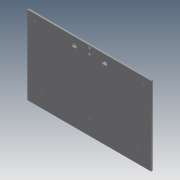
# Autodesk Inventor part: it bottom
Saved by Autodesk Inventor 2011 (Build 150239000, 239)
## iProperties
Created: 2011-09-03
Part Number: it bottom
Document SubType Name: Modeling
Designer: Matthew
Density: 1 g/cm^3
Author: Matthew
Autodesk Inventor part; units mm, degrees
ref_plane "YZ Plane" through (0, 0, 0) normal (1, 0, 0) x (0, 1, 0)
ref_plane "XZ Plane" through (0, 0, 0) normal (0, 1, 0) x (-1, 0, 0)
ref_plane "XY Plane" through (0, 0, 0) normal (0, 0, 1) x (1, 0, 0)
sketch "Sketch1" plane through (0, 0, 0) normal (0, 0, 1) x (1, 0, 0)
  line L0 (-37.7036, 22.272) -> (457.5964, 22.272)
  line L1 (457.5964, 22.272) -> (457.5964, -304.118)
  line L2 (457.5964, -304.118) -> (-37.7036, -304.118)
  line L3 (-37.7036, -304.118) -> (-37.7036, 22.272)
  point P0 (0, 0)
  dimension "d0" = 495.3
  dimension "d1" = 326.39
  constraints: 8 end point, 2 parallel, 1 horizontal, 1 perpendicular
  measures "d0" distance of L1.end L2.end
  measures "d1" distance of L0.end L1.end
extrude "Extrusion1" add sketch "Sketch1" along normal blind 6.35
sketch "Sketch2" plane through (0, 0, 6.35) normal (0, 0, 1) x (1, 0, 0)
  line L0 (-37.7036, 22.272) -> (457.5964, 22.272) projected
  line L1 (-37.7036, 22.272) -> (-18.6536, 22.272)
  line L2 (-18.6536, 22.272) -> (-18.6536, 15.922)
  line L3 (-18.6536, 15.922) -> (-37.7036, 15.922)
  line L4 (-37.7036, 15.922) -> (-37.7036, 22.272)
  line L5 (-18.6536, 15.922) -> (32.1464, 15.922)
  line L6 (32.1464, 15.922) -> (32.1464, 22.272)
  line L7 (32.1464, 22.272) -> (-18.6536, 22.272)
  line L8 (-18.6536, 22.272) -> (-18.6536, 15.922)
  line L9 (32.1464, 15.922) -> (82.9464, 15.922)
  line L10 (82.9464, 15.922) -> (82.9464, 22.272)
  line L11 (82.9464, 22.272) -> (32.1464, 22.272)
  line L12 (32.1464, 22.272) -> (32.1464, 15.922)
  line L13 (82.9464, 15.922) -> (133.7464, 15.922)
  line L14 (133.7464, 15.922) -> (133.7464, 22.272)
  line L15 (133.7464, 22.272) -> (82.9464, 22.272)
  line L16 (82.9464, 22.272) -> (82.9464, 15.922)
  line L17 (133.7464, 15.922) -> (184.5464, 15.922)
  line L18 (184.5464, 15.922) -> (184.5464, 22.272)
  line L19 (184.5464, 22.272) -> (133.7464, 22.272)
  line L20 (133.7464, 22.272) -> (133.7464, 15.922)
  line L21 (184.5464, 15.922) -> (235.3464, 15.922)
  line L22 (235.3464, 15.922) -> (235.3464, 22.272)
  line L23 (235.3464, 22.272) -> (184.5464, 22.272)
  line L24 (184.5464, 22.272) -> (184.5464, 15.922)
  line L25 (235.3464, 15.922) -> (286.1464, 15.922)
  line L26 (286.1464, 15.922) -> (286.1464, 22.272)
  line L27 (286.1464, 22.272) -> (235.3464, 22.272)
  line L28 (235.3464, 22.272) -> (235.3464, 15.922)
  line L29 (286.1464, 15.922) -> (336.9464, 15.922)
  line L30 (336.9464, 15.922) -> (336.9464, 22.272)
  line L31 (336.9464, 22.272) -> (286.1464, 22.272)
  line L32 (286.1464, 22.272) -> (286.1464, 15.922)
  line L33 (336.9464, 15.922) -> (387.7464, 15.922)
  line L34 (387.7464, 15.922) -> (387.7464, 22.272)
  line L35 (387.7464, 22.272) -> (336.9464, 22.272)
  line L36 (336.9464, 22.272) -> (336.9464, 15.922)
  line L37 (387.7464, 15.922) -> (438.5464, 15.922)
  line L38 (438.5464, 15.922) -> (438.5464, 22.272)
  line L39 (438.5464, 22.272) -> (387.7464, 22.272)
  line L40 (387.7464, 22.272) -> (387.7464, 15.922)
  line L41 (438.5464, 15.922) -> (457.5964, 15.922)
  line L42 (457.5964, 15.922) -> (457.5964, 22.272)
  line L43 (457.5964, 22.272) -> (438.5464, 22.272)
  line L44 (438.5464, 22.272) -> (438.5464, 15.922)
  point P0 (0, 0)
  dimension "d4" = 19.05
  dimension "d5" = 6.35
  dimension "d6" = 50.8
  dimension "d7" = 50.8
  dimension "d8" = 50.8
  dimension "d9" = 50.8
  dimension "d10" = 50.8
  dimension "d11" = 50.8
  dimension "d12" = 50.8
  dimension "d13" = 50.8
  dimension "d14" = 50.8
  constraints: 88 end point, 22 parallel, 11 horizontal, 11 perpendicular, 10 other
  measures "d4" distance of L2.end L3.end
  measures "d5" distance of L1.end L2.end
  measures "d6" distance of L7.end L6.end
  measures "d7" distance of L11.end L10.end
  measures "d8" distance of L15.end L14.end
  measures "d9" distance of L19.end L18.end
  measures "d10" distance of L23.end L22.end
  measures "d11" distance of L27.end L26.end
  measures "d12" distance of L31.end L30.end
  measures "d13" distance of L35.end L34.end
  measures "d14" distance of L39.end L38.end
extrude "Extrusion2" cut sketch "Sketch2" against normal blind 6.35 contours L0 L2 L3 L4 | L0 L10 L9 L6 | L0 L18 L17 L14 | L0 L26 L25 L22 | L0 L34 L33 L30 | L0 L42 L41 L38
sketch "Sketch3" plane through (0, 0, 6.35) normal (0, 0, 1) x (1, 0, 0)
  line L0 (457.5964, -304.118) -> (-37.7036, -304.118) projected
  line L1 (-37.7036, -304.118) -> (-18.6536, -304.118)
  line L2 (-18.6536, -304.118) -> (-18.6536, -297.768)
  line L3 (-18.6536, -297.768) -> (-37.7036, -297.768)
  line L4 (-37.7036, -297.768) -> (-37.7036, -304.118)
  line L5 (-18.6536, -297.768) -> (32.1464, -297.768)
  line L6 (32.1464, -297.768) -> (32.1464, -304.118)
  line L7 (32.1464, -304.118) -> (-18.6536, -304.118)
  line L8 (-18.6536, -304.118) -> (-18.6536, -297.768)
  line L9 (32.1464, -304.118) -> (82.9464, -304.118)
  line L10 (82.9464, -304.118) -> (82.9464, -297.768)
  line L11 (82.9464, -297.768) -> (32.1464, -297.768)
  line L12 (32.1464, -297.768) -> (32.1464, -304.118)
  line L13 (82.9464, -297.768) -> (133.7464, -297.768)
  line L14 (133.7464, -297.768) -> (133.7464, -304.118)
  line L15 (133.7464, -304.118) -> (82.9464, -304.118)
  line L16 (82.9464, -304.118) -> (82.9464, -297.768)
  line L17 (133.7464, -297.768) -> (184.5464, -297.768)
  line L18 (184.5464, -297.768) -> (184.5464, -304.118)
  line L19 (184.5464, -304.118) -> (133.7464, -304.118)
  line L20 (133.7464, -304.118) -> (133.7464, -297.768)
  line L21 (184.5464, -297.768) -> (235.3464, -297.768)
  line L22 (235.3464, -297.768) -> (235.3464, -304.118)
  line L23 (235.3464, -304.118) -> (184.5464, -304.118)
  line L24 (184.5464, -304.118) -> (184.5464, -297.768)
  line L25 (235.3464, -304.118) -> (286.1464, -304.118)
  line L26 (286.1464, -304.118) -> (286.1464, -297.768)
  line L27 (286.1464, -297.768) -> (235.3464, -297.768)
  line L28 (235.3464, -297.768) -> (235.3464, -304.118)
  line L29 (286.1464, -297.768) -> (336.9464, -297.768)
  line L30 (336.9464, -297.768) -> (336.9464, -304.118)
  line L31 (336.9464, -304.118) -> (286.1464, -304.118)
  line L32 (286.1464, -304.118) -> (286.1464, -297.768)
  line L33 (336.9464, -297.768) -> (387.7464, -297.768)
  line L34 (387.7464, -297.768) -> (387.7464, -304.118)
  line L35 (387.7464, -304.118) -> (336.9464, -304.118)
  line L36 (336.9464, -304.118) -> (336.9464, -297.768)
  line L37 (387.7464, -297.768) -> (438.5464, -297.768)
  line L38 (438.5464, -297.768) -> (438.5464, -304.118)
  line L39 (438.5464, -304.118) -> (387.7464, -304.118)
  line L40 (387.7464, -304.118) -> (387.7464, -297.768)
  line L41 (438.5464, -297.768) -> (457.5964, -297.768)
  line L42 (457.5964, -297.768) -> (457.5964, -304.118)
  line L43 (457.5964, -304.118) -> (438.5464, -304.118)
  line L44 (438.5464, -304.118) -> (438.5464, -297.768)
  point P0 (0, 0)
  dimension "d17" = 19.05
  dimension "d18" = 6.35
  constraints: 88 end point, 22 parallel, 11 horizontal, 11 perpendicular, 8 other
  measures "d17" distance of L3.end L2.end
  measures "d18" distance of L2.end L1.end
extrude "Extrusion3" cut sketch "Sketch3" against normal blind 6.35 contours L0 L38 L41 L42 | L0 L30 L33 L34 | L0 L14 L17 L18 | L0 L6 L11 L10 | L0 L4 L3 L2
sketch "Sketch4" plane through (0, 0, 6.35) normal (0, 0, 1) x (1, 0, 0)
  line L0 (336.9464, -304.118) -> (184.5464, -304.118) projected
  line L1 (184.5464, -304.118) -> (235.3464, -304.118)
  line L2 (235.3464, -304.118) -> (286.1464, -304.118)
  line L3 (286.1464, -304.118) -> (286.1464, -297.768)
  line L4 (286.1464, -297.768) -> (235.3464, -297.768)
  line L5 (235.3464, -297.768) -> (235.3464, -304.118)
  point P0 (0, 0)
  dimension "d21" = 50.8
  dimension "d22" = 50.8
  constraints: 10 end point, 2 parallel, 1 horizontal, 1 perpendicular, 1 point on line
  measures "d21" distance of L0.end L1.end
  measures "d22" distance of L4.end L3.end
extrude "Extrusion4" cut sketch "Sketch4" against normal blind 6.35
sketch "Sketch5" plane through (0, 0, 6.35) normal (0, 0, 1) x (1, 0, 0)
  line L0 (457.5964, 15.922) -> (457.5964, -297.768) projected
  line L1 (-37.7036, -297.768) -> (-37.7036, 15.922) projected
  line L2 (-37.7036, -297.768) -> (-18.6536, -297.768) projected
  line L3 (457.5964, 15.922) -> (457.5964, -166.323)
  line L4 (457.5964, -166.323) -> (451.2464, -166.323)
  line L5 (451.2464, -166.323) -> (451.2464, -115.523)
  line L6 (451.2464, -115.523) -> (457.5964, -115.523)
  line L7 (457.5964, -115.523) -> (457.5964, -166.323)
  line L8 (451.2464, -115.523) -> (457.5964, -115.523)
  line L9 (457.5964, -115.523) -> (457.5964, -64.723)
  line L10 (457.5964, -64.723) -> (451.2464, -64.723)
  line L11 (451.2464, -64.723) -> (451.2464, -115.523)
  line L12 (451.2464, -64.723) -> (457.5964, -64.723)
  line L13 (457.5964, -64.723) -> (457.5964, -13.923)
  line L14 (457.5964, -13.923) -> (451.2464, -13.923)
  line L15 (451.2464, -13.923) -> (451.2464, -64.723)
  line L16 (451.2464, -166.323) -> (457.5964, -166.323)
  line L17 (457.5964, -166.323) -> (457.5964, -217.123)
  line L18 (457.5964, -217.123) -> (451.2464, -217.123)
  line L19 (451.2464, -217.123) -> (451.2464, -166.323)
  line L20 (451.2464, -217.123) -> (457.5964, -217.123)
  line L21 (457.5964, -217.123) -> (457.5964, -267.923)
  line L22 (457.5964, -267.923) -> (451.2464, -267.923)
  line L23 (451.2464, -267.923) -> (451.2464, -217.123)
  line L24 (451.2464, -267.923) -> (457.5964, -267.923)
  line L25 (457.5964, -267.923) -> (457.5964, -297.768)
  line L26 (457.5964, -297.768) -> (451.2464, -297.768)
  line L27 (451.2464, -297.768) -> (451.2464, -267.923)
  line L28 (451.2464, -13.923) -> (457.5964, -13.923)
  line L29 (457.5964, -13.923) -> (457.5964, 15.922)
  line L30 (457.5964, 15.922) -> (451.2464, 15.922)
  line L31 (451.2464, 15.922) -> (451.2464, -13.923)
  line L32 (-37.7036, 15.922) -> (-31.3536, 15.922)
  line L33 (-31.3536, 15.922) -> (-31.3536, -13.923)
  line L34 (-31.3536, -13.923) -> (-37.7036, -13.923)
  line L35 (-37.7036, -13.923) -> (-37.7036, 15.922)
  line L36 (-37.7036, -64.723) -> (-31.3536, -64.723)
  line L37 (-31.3536, -64.723) -> (-31.3536, -115.523)
  line L38 (-31.3536, -115.523) -> (-37.7036, -115.523)
  line L39 (-37.7036, -115.523) -> (-37.7036, -64.723)
  line L40 (-37.7036, -166.323) -> (-31.3536, -166.323)
  line L41 (-31.3536, -166.323) -> (-31.3536, -217.123)
  line L42 (-31.3536, -217.123) -> (-37.7036, -217.123)
  line L43 (-37.7036, -217.123) -> (-37.7036, -166.323)
  line L44 (-37.7036, -267.923) -> (-31.3536, -267.923)
  line L45 (-31.3536, -267.923) -> (-31.3536, -297.768)
  line L46 (-31.3536, -297.768) -> (-37.7036, -297.768)
  line L47 (-37.7036, -297.768) -> (-37.7036, -267.923)
  point P0 (0, 0)
  dimension "d25" = 182.245
  dimension "d26" = 6.35
  dimension "d27" = 50.8
  dimension "d28" = 50.8
  dimension "d29" = 50.8
  dimension "d30" = 50.8
  dimension "d31" = 50.8
  dimension "d32" = 6.35
  constraints: 90 end point, 22 parallel, 11 horizontal, 11 perpendicular, 9 point on line
  measures "d25" distance of L0.start L3.end
  measures "d26" distance of L5.end L6.end
  measures "d27" distance of L4.end L5.end
  measures "d28" distance of L9.end L8.end
  measures "d29" distance of L13.end L12.end
  measures "d30" distance of L16.end L17.end
  measures "d31" distance of L20.end L21.end
  measures "d32" distance of L33.end L34.end
extrude "Extrusion5" cut sketch "Sketch5" against normal blind 6.35 contours L0 L14 L31 L30 | L0 L18 L19 L4 | L0 L26 L27 L22 | L1 L44 L45 L2 | L1 L40 L41 L42 | L1 L36 L37 L38 | L1 L32 L33 L34
sketch "Sketch6" plane through (0, 0, 6.35) normal (0, 0, 1) x (1, 0, 0)
  line L0 (457.5964, -13.923) -> (457.5964, -166.323) projected
  line L1 (457.5964, -13.923) -> (457.5964, -64.723)
  line L2 (457.5964, -64.723) -> (451.2464, -64.723)
  line L3 (451.2464, -64.723) -> (451.2464, -115.523)
  line L4 (451.2464, -115.523) -> (457.5964, -115.523)
  line L5 (457.5964, -115.523) -> (457.5964, -64.723)
  point P0 (0, 0)
  constraints: 10 end point, 2 parallel, 1 horizontal, 1 perpendicular, 1 point on line
extrude "Extrusion6" cut sketch "Sketch6" against normal blind 6.35
sketch "Sketch7" plane through (0, 0, 6.35) normal (0, 0, 1) x (1, 0, 0)
  line L0 (451.2464, -13.923) -> (451.2464, 15.922) projected
  line L1 (387.7464, 15.922) -> (336.9464, 15.922) projected
  line L2 (82.9464, 15.922) -> (32.1464, 15.922) projected
  line L3 (-31.3536, 15.922) -> (-31.3536, -13.923) projected
  line L4 (451.2464, -115.523) -> (451.2464, -64.723) projected
  line L5 (-31.3536, -6.7444) -> (44.8464, -6.7444)
  line L6 (44.8464, -6.7444) -> (44.8464, 15.922)
  line L7 (44.8464, 15.922) -> (44.8464, -60.278)
  line L8 (451.2464, -6.7444) -> (375.0464, -6.7444)
  line L9 (375.0464, -6.7444) -> (375.0464, 15.922)
  line L10 (375.0464, 15.922) -> (375.0464, -60.278)
  circle A0 centre (44.8464, -60.278) radius 25.4
  circle A1 centre (375.0464, -60.278) radius 25.4
  point P0 (0, 0)
  dimension "d37" = 76.2
  dimension "d38" = 76.2
  dimension "d39" = 76.2
  dimension "d40" = 76.2
  dimension "d41" = 50.8
  dimension "d42" = 50.8
  constraints: 12 end point, 4 perpendicular, 4 point on line, 2 centre point, 2 coincident, 2 collinear
  measures "d37" distance of L5.start L5.end
  measures "d38" distance of L6.end L7.end
  measures "d39" distance of L8.start L8.end
  measures "d40" distance of L9.end L10.end
  measures "d41" diameter of A0
  measures "d42" diameter of A1
extrude "Extrusion7" cut sketch "Sketch7" against normal blind 25.4
sketch "Sketch8" plane through (0, 0, 6.35) normal (0, 0, 1) x (1, 0, 0)
  line L0 (-31.3536, -297.768) -> (-37.7036, -297.768)
  line L1 (-37.7036, -297.768) -> (-37.7036, 15.922)
  line L2 (-37.7036, 15.922) -> (-31.3536, 15.922)
  line L3 (-31.3536, 15.922) -> (-31.3536, -297.768)
  point P0 (0, 0)
  constraints: 8 end point, 2 parallel, 1 horizontal, 1 perpendicular
extrude "Extrusion8" add sketch "Sketch8" against normal blind 6.35
sketch "Sketch9" plane through (0, 0, 6.35) normal (0, 0, 1) x (1, 0, 0)
  line L0 (451.2464, -297.768) -> (457.5964, -297.768)
  line L1 (457.5964, -297.768) -> (457.5964, 15.922)
  line L2 (457.5964, 15.922) -> (451.2464, 15.922)
  line L3 (451.2464, 15.922) -> (451.2464, -297.768)
  point P0 (0, 0)
  constraints: 8 end point, 2 parallel, 1 horizontal, 1 perpendicular
extrude "Extrusion9" add sketch "Sketch9" against normal blind 6.35
sketch "Sketch10" plane through (0, 0, 6.35) normal (0, 0, 1) x (1, 0, 0)
  line L0 (457.5964, 15.922) -> (438.5464, 15.922) projected
  line L1 (438.5464, 15.922) -> (438.5464, 22.272) projected
  line L2 (387.7464, 22.272) -> (438.5464, 22.272) projected
  line L3 (387.7464, 22.272) -> (387.7464, 15.922) projected
  line L4 (387.7464, 15.922) -> (336.9464, 15.922) projected
  line L5 (336.9464, 15.922) -> (336.9464, 22.272) projected
  line L6 (286.1464, 22.272) -> (336.9464, 22.272) projected
  line L7 (286.1464, 22.272) -> (286.1464, 15.922) projected
  line L8 (286.1464, 15.922) -> (235.3464, 15.922) projected
  line L9 (235.3464, 15.922) -> (235.3464, 22.272) projected
  line L10 (184.5464, 22.272) -> (235.3464, 22.272) projected
  line L11 (184.5464, 22.272) -> (184.5464, 15.922) projected
  line L12 (184.5464, 15.922) -> (133.7464, 15.922) projected
  line L13 (133.7464, 15.922) -> (133.7464, 22.272) projected
  line L14 (82.9464, 22.272) -> (133.7464, 22.272) projected
  line L15 (82.9464, 22.272) -> (82.9464, 15.922) projected
  line L16 (82.9464, 15.922) -> (32.1464, 15.922) projected
  line L17 (32.1464, 15.922) -> (32.1464, 22.272) projected
  line L18 (-18.6536, 22.272) -> (32.1464, 22.272) projected
  line L19 (-18.6536, 22.272) -> (-18.6536, 15.922) projected
  line L20 (-18.6536, 15.922) -> (-37.7036, 15.922) projected
  line L21 (-37.7036, 15.922) -> (-37.7036, -297.768) projected
  line L22 (-37.7036, -297.768) -> (-18.6536, -297.768) projected
  line L23 (-18.6536, -297.768) -> (-18.6536, -304.118) projected
  line L24 (32.1464, -304.118) -> (-18.6536, -304.118) projected
  line L25 (32.1464, -304.118) -> (32.1464, -297.768) projected
  line L26 (32.1464, -297.768) -> (82.9464, -297.768) projected
  line L27 (82.9464, -297.768) -> (82.9464, -304.118) projected
  line L28 (133.7464, -304.118) -> (82.9464, -304.118) projected
  line L29 (133.7464, -304.118) -> (133.7464, -297.768) projected
  line L30 (133.7464, -297.768) -> (184.5464, -297.768) projected
  line L31 (184.5464, -297.768) -> (184.5464, -304.118) projected
  line L32 (235.3464, -304.118) -> (184.5464, -304.118) projected
  line L33 (235.3464, -304.118) -> (235.3464, -297.768) projected
  line L34 (235.3464, -297.768) -> (286.1464, -297.768) projected
  line L35 (286.1464, -297.768) -> (286.1464, -304.118) projected
  line L36 (336.9464, -304.118) -> (286.1464, -304.118) projected
  line L37 (336.9464, -304.118) -> (336.9464, -297.768) projected
  line L38 (336.9464, -297.768) -> (387.7464, -297.768) projected
  line L39 (387.7464, -297.768) -> (387.7464, -304.118) projected
  line L40 (438.5464, -304.118) -> (387.7464, -304.118) projected
  line L41 (438.5464, -304.118) -> (438.5464, -297.768) projected
  line L42 (438.5464, -297.768) -> (457.5964, -297.768) projected
  line L43 (457.5964, 15.922) -> (457.5964, -297.768) projected
  line L44 (-18.6536, -297.768) -> (438.5464, -297.768)
  line L45 (438.5464, 15.922) -> (-18.6536, 15.922)
  point P0 (0, 0)
  constraints: 4 end point, 1 parallel, 1 perpendicular
extrude "Extrusion10" cut sketch "Sketch10" against normal blind 6.35 contours L45 L3 L2 L1 | L41 L40 L39 L44 | L45 L7 L6 L5 | L37 L36 L35 L44 | L45 L11 L10 L9 | L33 L32 L31 L44 | L45 L15 L14 L13 | L29 L28 L27 L44 | L45 L19 L18 L17 | L25 L24 L23 L44
sketch "Sketch12" plane through (0, 0, 6.35) normal (0, 0, 1) x (1, 0, 0)
  circle A0 centre (44.8464, -60.278) radius 25.4 projected
  circle A1 centre (375.0464, -60.278) radius 25.4 projected
  point P0 (0, 0)
extrude "Extrusion11" add sketch "Sketch12" against normal blind 6.35
sketch "Sketch13" plane through (0, 0, 6.35) normal (0, 0, 1) x (1, 0, 0)
  line L0 (457.5964, 15.922) -> (-37.7036, 15.922) projected
  line L1 (-37.7036, 15.922) -> (-37.7036, -297.768) projected
  line L2 (457.5964, 15.922) -> (368.6964, 15.922)
  line L3 (368.6964, 15.922) -> (368.6964, -66.628)
  line L4 (-37.7036, -66.628) -> (44.8464, -66.628)
  circle A0 centre (368.6964, -66.628) radius 25.4
  circle A1 centre (44.8464, -66.628) radius 25.4
  point P0 (0, 0)
  dimension "d53" = 88.9
  dimension "d54" = 82.55
  dimension "d55" = 82.55
  dimension "d56" = 50.8
  dimension "d57" = 50.8
  constraints: 6 end point, 2 centre point, 2 coincident, 2 perpendicular, 2 point on line
  measures "d53" distance of L0.start L2.end
  measures "d54" distance of L2.end L3.end
  measures "d55" distance of L4.start L4.end
  measures "d56" diameter of A0
  measures "d57" diameter of A1
extrude "Extrusion12" cut sketch "Sketch13" against normal blind 6.35
sketch "Sketch14" plane through (0, 0, 6.35) normal (0, 0, 1) x (1, 0, 0)
  circle A0 centre (368.6964, -66.628) radius 25.4 projected
  circle A1 centre (44.8464, -66.628) radius 25.4 projected
  point P0 (0, 0)
extrude "Extrusion13" add sketch "Sketch14" against normal blind 6.35
sketch "Sketch15" plane through (0, 0, 6.35) normal (0, 0, 1) x (1, 0, 0)
  line L0 (457.5964, 15.922) -> (375.0464, 15.922)
  line L1 (375.0464, 15.922) -> (375.0464, -71.4032)
  line L2 (375.0464, -71.4032) -> (457.5964, -71.4032)
  line L3 (457.5964, -71.4032) -> (457.5964, 15.922)
  line L4 (-37.7036, 15.922) -> (44.8464, 15.922)
  line L5 (44.8464, 15.922) -> (44.8464, -71.4032)
  line L6 (44.8464, -71.4032) -> (-37.7036, -71.4032)
  line L7 (-37.7036, -71.4032) -> (-37.7036, 15.922)
  circle A0 centre (375.0464, -71.4032) radius 25.4
  circle A1 centre (44.8464, -71.4032) radius 25.4
  point P0 (0, 0)
  dimension "d62" = 82.55
  dimension "d63" = 87.3252
  dimension "d64" = 82.55
  dimension "d65" = 87.3252
  dimension "d66" = 50.8
  dimension "d67" = 50.8
  constraints: 16 end point, 4 parallel, 2 centre point, 2 coincident, 2 horizontal, 2 perpendicular
  measures "d62" distance of L2.end L1.end
  measures "d63" distance of L1.end L0.end
  measures "d64" distance of L5.end L6.end
  measures "d65" distance of L4.end L5.end
  measures "d66" diameter of A0
  measures "d67" diameter of A1
extrude "Extrusion14" cut sketch "Sketch15" against normal blind 6.35 contours A0 L2 L1 | L1 L2 A0 | A1 L6 L5 | L5 L6 A1
sketch "Sketch16" plane through (0, 0, 6.35) normal (0, 0, 1) x (1, 0, 0)
  line L0 (-37.7036, 15.922) -> (-5.9536, 15.922)
  line L1 (-5.9536, 15.922) -> (-5.9536, -9.478)
  line L2 (-5.9536, -9.478) -> (-37.7036, -9.478)
  line L3 (-37.7036, -9.478) -> (-37.7036, 15.922)
  line L4 (-37.7036, -297.768) -> (19.4464, -297.768)
  line L5 (19.4464, -297.768) -> (19.4464, -240.618)
  line L6 (19.4464, -240.618) -> (-37.7036, -240.618)
  line L7 (-37.7036, -240.618) -> (-37.7036, -297.768)
  line L8 (457.5964, 15.922) -> (425.8464, 15.922)
  line L9 (425.8464, 15.922) -> (425.8464, -9.478)
  line L10 (425.8464, -9.478) -> (457.5964, -9.478)
  line L11 (457.5964, -9.478) -> (457.5964, 15.922)
  line L12 (457.5964, -297.768) -> (400.4464, -297.768)
  line L13 (400.4464, -297.768) -> (400.4464, -240.618)
  line L14 (400.4464, -240.618) -> (457.5964, -240.618)
  line L15 (457.5964, -240.618) -> (457.5964, -297.768)
  circle A0 centre (400.4464, -240.618) radius 1.9812
  circle A1 centre (19.4464, -240.618) radius 1.9812
  circle A2 centre (-5.9536, -9.478) radius 1.9812
  circle A3 centre (425.8464, -9.478) radius 1.9812
  point P0 (0, 0)
  dimension "d70" = 31.75
  dimension "d71" = 25.4
  dimension "d72" = 57.15
  dimension "d73" = 57.15
  dimension "d74" = 31.75
  dimension "d75" = 57.15
  dimension "d76" = 3.9624
  dimension "d77" = 3.9624
  dimension "d78" = 3.9624
  dimension "d79" = 3.9624
  constraints: 32 end point, 8 parallel, 4 centre point, 4 coincident, 4 horizontal, 4 perpendicular
  measures "d70" distance of L1.end L2.end
  measures "d71" distance of L0.end L1.end
  measures "d72" distance of L6.end L5.end
  measures "d73" distance of L5.end L4.end
  measures "d74" distance of L10.end L9.end
  measures "d75" distance of L13.end L14.end
  measures "d76" diameter of A0
  measures "d77" diameter of A1
  measures "d78" diameter of A2
  measures "d79" diameter of A3
extrude "Extrusion15" cut sketch "Sketch16" against normal blind 25.4 contours A2 L2 L1 | L1 L2 A2 | A3 L10 L9 | L9 L10 A3
sketch "Sketch17" plane through (0, 0, 6.35) normal (0, 0, 1) x (1, 0, 0)
  circle A0 centre (425.8464, -9.478) radius 1.9812 projected
  line L0 (457.5964, 15.922) -> (457.5964, -297.768) projected
  line L1 (425.8464, -9.478) -> (425.8464, -272.368)
  line L2 (425.8464, -272.368) -> (0, -272.368)
  line L3 (0, -272.368) -> (25.4, -272.368)
  line L4 (25.4, -272.368) -> (25.4, -246.968)
  line L5 (425.8464, -246.968) -> (400.4464, -246.968)
  circle A1 centre (400.4464, -246.968) radius 1.9812
  circle A2 centre (25.4, -246.968) radius 1.9812
  point P0 (0, 0)
  dimension "d82" = 262.89
  dimension "d83" = 25.4
  dimension "d84" = 25.4
  dimension "d85" = 25.4
  dimension "d86" = 3.9624
  dimension "d87" = 3.9624
  constraints: 10 end point, 3 perpendicular, 2 centre point, 2 coincident, 2 point on line, 1 parallel
  measures "d82" distance of L1.start L1.end
  measures "d83" distance of L2.end L3.end
  measures "d84" distance of L3.end L4.end
  measures "d85" distance of L5.start L5.end
  measures "d86" diameter of A1
  measures "d87" diameter of A2
extrude "Extrusion16" cut sketch "Sketch17" against normal blind 25.4 contours A1 | A2
sketch "Sketch18" plane through (0, 0, 6.35) normal (0, 0, 1) x (1, 0, 0)
  circle A0 centre (25.4, -246.968) radius 1.9812 projected
  point P0 (0, 0)
extrude "Extrusion17" add sketch "Sketch18" against normal blind 6.35
sketch "Sketch19" plane through (0, 0, 6.35) normal (0, 0, 1) x (1, 0, 0)
  circle A0 centre (-5.9536, -9.478) radius 1.9812 projected
  line L0 (457.5964, 15.922) -> (457.5964, -297.768) projected
  line L1 (-5.9536, -9.478) -> (-5.9536, -272.368)
  line L2 (-5.9536, -272.368) -> (19.4464, -272.368)
  line L3 (19.4464, -272.368) -> (19.4464, -246.968)
  circle A1 centre (19.4464, -246.968) radius 1.9812
  point P0 (0, 0)
  dimension "d92" = 262.89
  dimension "d93" = 25.4
  dimension "d94" = 25.4
  dimension "d95" = 3.9624
  constraints: 6 end point, 2 parallel, 1 centre point, 1 coincident, 1 perpendicular
  measures "d92" distance of L1.start L1.end
  measures "d93" distance of L1.end L2.end
  measures "d94" distance of L2.end L3.end
  measures "d95" diameter of A1
extrude "Extrusion18" cut sketch "Sketch19" against normal blind 6.35 contours A1
sketch "Sketch20" plane through (0, 0, 0) normal (0, 0, -1) x (-1, 0, 0)
  line L0 (37.7036, 15.922) -> (-457.5964, 15.922) projected
  line L1 (37.7036, 15.922) -> (37.7036, -297.768) projected
  line L2 (-209.9464, 15.922) -> (-209.9464, 7.922)
  line L3 (-209.9464, 15.922) -> (-209.9464, -14.078)
  circle A0 centre (-209.9464, 7.922) radius 5
  circle A1 centre (-209.9464, -14.078) radius 5
  point P0 (0, 0)
  dimension "d98" = 8
  dimension "d99" = 30
  dimension "d100" = 10
  dimension "d101" = 10
  constraints: 4 end point, 2 centre point, 2 coincident, 1 midpoint, 1 parallel, 1 point on line
  measures "d98" distance of L2.start L2.end
  measures "d99" distance of L2.start L3.end
  measures "d100" diameter of A0
  measures "d101" diameter of A1
extrude "Extrusion19" cut sketch "Sketch20" against normal blind 6.35
sketch "Sketch21" plane through (0, 0, 6.35) normal (0, 0, 1) x (1, 0, 0)
  line L0 (457.5964, 15.922) -> (-37.7036, 15.922) projected
  line L1 (457.5964, 15.922) -> (457.5964, -297.768) projected
  line L2 (209.9464, 15.922) -> (209.9464, -22.178)
  line L3 (209.9464, -22.178) -> (235.3464, -22.178)
  line L4 (235.3464, -22.178) -> (184.5464, -22.178)
  line L5 (235.3464, -22.178) -> (260.7464, -22.178)
  line L6 (184.5464, -22.178) -> (159.1464, -22.178)
  line L7 (260.7464, -22.178) -> (279.7964, -22.178)
  line L8 (279.7964, -22.178) -> (279.7964, -9.478)
  line L9 (279.7964, -9.478) -> (260.7464, -9.478)
  line L10 (260.7464, -9.478) -> (260.7464, -22.178)
  line L11 (159.1464, -22.178) -> (140.0964, -22.178)
  line L12 (140.0964, -22.178) -> (140.0964, -9.478)
  line L13 (140.0964, -9.478) -> (159.1464, -9.478)
  line L14 (159.1464, -9.478) -> (159.1464, -22.178)
  point P0 (0, 0)
  dimension "d104" = 38.1
  dimension "d105" = 25.4
  dimension "d106" = 50.8
  dimension "d107" = 25.4
  dimension "d108" = 25.4
  dimension "d109" = 19.05
  dimension "d110" = 12.7
  dimension "d111" = 19.05
  dimension "d112" = 12.7
  constraints: 26 end point, 5 parallel, 3 collinear, 3 perpendicular, 2 horizontal, 1 midpoint
  measures "d104" distance of L2.start L2.end
  measures "d105" distance of L2.end L3.end
  measures "d106" distance of L3.end L4.end
  measures "d107" distance of L3.end L5.end
  measures "d108" distance of L4.end L6.end
  measures "d109" distance of L9.end L8.end
  measures "d110" distance of L8.end L7.end
  measures "d111" distance of L12.end L13.end
  measures "d112" distance of L11.end L12.end
extrude "Extrusion20" cut sketch "Sketch21" against normal blind 6.35
sketch "Sketch22" plane through (0, 0, 6.35) normal (0, 0, 1) x (1, 0, 0)
  line L0 (457.5964, 15.922) -> (-37.7036, 15.922) projected
  line L1 (457.5964, 15.922) -> (457.5964, -297.768) projected
  line L2 (209.9464, 15.922) -> (209.9464, -240.745)
  circle A0 centre (209.9464, -240.745) radius 1.9812
  point P0 (0, 0)
  dimension "d115" = 256.667
  dimension "d116" = 3.9624
  constraints: 2 end point, 1 centre point, 1 coincident, 1 midpoint, 1 parallel
  measures "d115" distance of L2.start L2.end
  measures "d116" diameter of A0
extrude "Extrusion21" cut sketch "Sketch22" against normal blind 6.35
sketch "Sketch23" plane through (0, 0, 6.35) normal (0, 0, 1) x (1, 0, 0)
  circle A0 centre (375.0464, -71.4032) radius 25.4 projected
  circle A1 centre (44.8464, -71.4032) radius 25.4 projected
  point P0 (0, 0)
extrude "Extrusion22" add sketch "Sketch23" against normal blind 6.35
sketch "Sketch24" plane through (0, 0, 6.35) normal (0, 0, 1) x (1, 0, 0)
  line L0 (457.5964, 15.922) -> (375.0464, 15.922)
  line L1 (375.0464, 15.922) -> (375.0464, -72.978)
  line L2 (375.0464, -72.978) -> (457.5964, -72.978)
  line L3 (457.5964, -72.978) -> (457.5964, 15.922)
  line L4 (-37.7036, 15.922) -> (44.8464, 15.922)
  line L5 (44.8464, 15.922) -> (44.8464, -72.978)
  line L6 (44.8464, -72.978) -> (-37.7036, -72.978)
  line L7 (-37.7036, -72.978) -> (-37.7036, 15.922)
  circle A0 centre (375.0464, -72.978) radius 25.4
  circle A1 centre (44.8464, -72.978) radius 25.4
  point P0 (0, 0)
  dimension "d121" = 82.55
  dimension "d122" = 88.9
  dimension "d123" = 82.55
  dimension "d124" = 50.8
  dimension "d125" = 50.8
  constraints: 16 end point, 4 parallel, 2 centre point, 2 coincident, 2 horizontal, 2 perpendicular
  measures "d121" distance of L2.end L1.end
  measures "d122" distance of L1.end L0.end
  measures "d123" distance of L5.end L6.end
  measures "d124" diameter of A0
  measures "d125" diameter of A1
extrude "Extrusion23" cut sketch "Sketch24" against normal blind 6.35 contours A0 L2 L1 | L1 L2 A0 | A1 L6 L5 | L5 L6 A1
body "Solid1"
